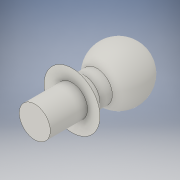
# Autodesk Inventor part: Ball-Joint-male
Saved by Autodesk Inventor 2018.2 (Build 222227000, 227)
## iProperties
Created: 2018-02-18
Part Number: Ball-Joint-male
Material: Generisch
Document SubType Name: Modeling
Designer: JochenAlt
Density: 1 g/cm^3
Appearance: Vorgabe
Author: JochenAlt
Autodesk Inventor part; units mm, degrees
ref_plane "YZ Plane" through (0, 0, 0) normal (1, 0, 0) x (0, 1, 0)
ref_plane "XZ Plane" through (0, 0, 0) normal (0, 1, 0) x (-1, 0, 0)
ref_plane "XY Plane" through (0, 0, 0) normal (0, 0, 1) x (1, 0, 0)
sketch "Skizze1" plane through (0, 0, 0) normal (0, 0, 1) x (1, 0, 0)
  line L0 (-0.5345, 0) -> (3.2068, 0) construction
  line L1 (0, 11.2263) -> (0, -1.8711) construction
  line L2 (0, 0) -> (1.25, 0)
  line L3 (1.25, 3) -> (1.25, 0)
  line L4 (1.25, 3) -> (2.25, 3)
  line L5 (2.25, 3) -> (1.25, 4)
  line L6 (1.25, 4) -> (1.25, 5)
  arc A0 (1.25, 5) -> (0, 8.8993) centre (0, 6.7493) ccw
  line L7 (0, 8.8993) -> (0, 0)
  dimension "d0" = 4.3
  dimension "d1" = 1.25
  dimension "d2" = 3
  dimension "d3" = 1
  dimension "d4" = 1
  dimension "d6" = 1
  constraints: 12 end point, 4 point on line, 2 point on circle, 1 centre point, 1 collinear, 1 horizontal, 1 perpendicular
  measures "d0" diameter of A0
  measures "d1" distance between parallel lines of L1 L3
  measures "d2" distance between parallel lines of L0 L4
  measures "d3" distance from line of L4 L5.end
  measures "d4" distance of L6.end L5.end
  measures "d6" distance of L4.end L3.start
revolve "Umdrehung1" add sketch "Skizze1" angle 360 about axis through (0, 0, 0) along (0, -1, 0)
